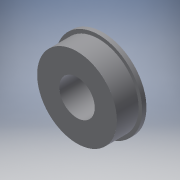
# Autodesk Inventor part: bearing
Saved by Autodesk Inventor 2016 (Build 200138000, 138)
## iProperties
Created: 2016-01-17
Part Number: bearing
Material: Generic
Document SubType Name: Modeling
Designer: gus
Mass: 4.96563 g
Surface Area: 24.8502 cm^2
Volume: 4.96563 cm^3
Density: 1 g/cm^3
Appearance: Default
User Status: have
Author: gus
Autodesk Inventor part; units mm, degrees
ref_plane "YZ Plane" through (0, 0, 0) normal (1, 0, 0) x (0, 1, 0)
ref_plane "XZ Plane" through (0, 0, 0) normal (0, 1, 0) x (-1, 0, 0)
ref_plane "XY Plane" through (0, 0, 0) normal (0, 0, 1) x (1, 0, 0)
sketch "Sketch1" plane through (0, 0, 0) normal (0, 0, 1) x (1, 0, 0)
  circle A0 centre (0, 0) radius 14.2875
  circle A1 centre (0, 0) radius 6.35
  dimension "d0" = 28.575
  dimension "d1" = 12.7
  constraints: 2 centre point, 2 coincident
  measures "d0" diameter of A0
  measures "d1" diameter of A1
extrude "Extrusion1" add sketch "Sketch1" along normal blind 7.7724
sketch "Sketch2" plane through (0, 0, 0) normal (0, 0, -1) x (-1, 0, 0)
  circle A0 centre (0, 0) radius 15.5575
  circle A1 centre (0, 0) radius 14.2875 projected
  circle A2 centre (0, 0) radius 6.35
  dimension "d4" = 31.115
  dimension "d5" = 12.7
  constraints: 2 centre point, 2 coincident
  measures "d4" diameter of A0
  measures "d5" diameter of A2
extrude "Extrusion2" add sketch "Sketch2" along normal blind 1.524 contours A0 | A1
body "Solid1"
